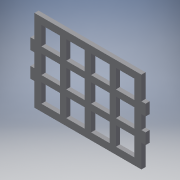
# Autodesk Inventor part: Top
Saved by Autodesk Inventor 2018 (Build 220112000, 112)
## iProperties
Created: 2017-10-30
Part Number: Top
Material: Polycarbonate, Clear
Document SubType Name: Modeling
Designer: xl0
Density: 1.2 g/cm^3
Appearance: Polycarbonate - Clear
Author: xl0
Autodesk Inventor part; units mm, degrees
ref_plane "YZ Plane" through (0, 0, 0) normal (1, 0, 0) x (0, 1, 0)
ref_plane "XZ Plane" through (0, 0, 0) normal (0, 1, 0) x (-1, 0, 0)
ref_plane "XY Plane" through (0, 0, 0) normal (0, 0, 1) x (1, 0, 0)
sketch "Sketch1" plane through (0, 0, 0) normal (0, 0, 1) x (1, 0, 0)
  line L0 (-38.75, 29.75) -> (38.75, 29.75)
  line L1 (38.75, 29.75) -> (38.75, -29.75)
  line L2 (38.75, -29.75) -> (-38.75, -29.75)
  line L3 (-38.75, -29.75) -> (-38.75, 29.75)
  line L4 (-33.75, 24.75) -> (-20.25, 24.75)
  line L5 (-20.25, 24.75) -> (-20.25, 11.25)
  line L6 (-20.25, 11.25) -> (-33.75, 11.25)
  line L7 (-33.75, 11.25) -> (-33.75, 24.75)
  line L8 (-2.25, 24.75) -> (-2.25, 11.25)
  line L9 (-15.75, 24.75) -> (-2.25, 24.75)
  line L10 (-15.75, 11.25) -> (-15.75, 24.75)
  line L11 (-2.25, 11.25) -> (-15.75, 11.25)
  line L12 (15.75, 24.75) -> (15.75, 11.25)
  line L13 (2.25, 24.75) -> (15.75, 24.75)
  line L14 (2.25, 11.25) -> (2.25, 24.75)
  line L15 (15.75, 11.25) -> (2.25, 11.25)
  line L16 (33.75, 24.75) -> (33.75, 11.25)
  line L17 (20.25, 24.75) -> (33.75, 24.75)
  line L18 (20.25, 11.25) -> (20.25, 24.75)
  line L19 (33.75, 11.25) -> (20.25, 11.25)
  line L20 (-20.25, 6.75) -> (-20.25, -6.75)
  line L21 (-33.75, 6.75) -> (-20.25, 6.75)
  line L22 (-33.75, -6.75) -> (-33.75, 6.75)
  line L23 (-20.25, -6.75) -> (-33.75, -6.75)
  line L24 (-2.25, 6.75) -> (-2.25, -6.75)
  line L25 (-15.75, 6.75) -> (-2.25, 6.75)
  line L26 (-15.75, -6.75) -> (-15.75, 6.75)
  line L27 (-2.25, -6.75) -> (-15.75, -6.75)
  line L28 (15.75, 6.75) -> (15.75, -6.75)
  line L29 (2.25, 6.75) -> (15.75, 6.75)
  line L30 (2.25, -6.75) -> (2.25, 6.75)
  line L31 (15.75, -6.75) -> (2.25, -6.75)
  line L32 (33.75, 6.75) -> (33.75, -6.75)
  line L33 (20.25, 6.75) -> (33.75, 6.75)
  line L34 (20.25, -6.75) -> (20.25, 6.75)
  line L35 (33.75, -6.75) -> (20.25, -6.75)
  line L36 (-20.25, -11.25) -> (-20.25, -24.75)
  line L37 (-33.75, -11.25) -> (-20.25, -11.25)
  line L38 (-33.75, -24.75) -> (-33.75, -11.25)
  line L39 (-20.25, -24.75) -> (-33.75, -24.75)
  line L40 (-2.25, -11.25) -> (-2.25, -24.75)
  line L41 (-15.75, -11.25) -> (-2.25, -11.25)
  line L42 (-15.75, -24.75) -> (-15.75, -11.25)
  line L43 (-2.25, -24.75) -> (-15.75, -24.75)
  line L44 (15.75, -11.25) -> (15.75, -24.75)
  line L45 (2.25, -11.25) -> (15.75, -11.25)
  line L46 (2.25, -24.75) -> (2.25, -11.25)
  line L47 (15.75, -24.75) -> (2.25, -24.75)
  line L48 (33.75, -11.25) -> (33.75, -24.75)
  line L49 (20.25, -11.25) -> (33.75, -11.25)
  line L50 (20.25, -24.75) -> (20.25, -11.25)
  line L51 (33.75, -24.75) -> (20.25, -24.75)
  line L52 (-38.75, 13) -> (-41.75, 13)
  line L53 (-41.75, 13) -> (-41.75, 5)
  line L54 (-41.75, 5) -> (-38.75, 5)
  line L55 (-38.75, -5) -> (-41.75, -5)
  line L56 (-41.75, -5) -> (-41.75, -13)
  line L57 (-41.75, -13) -> (-38.75, -13)
  line L58 (-22.2351, 9) -> (-45.0452, 9) construction
  line L59 (-22.7359, -9) -> (-44.2257, -9) construction
  line L60 (38.75, 13) -> (41.75, 13)
  line L61 (41.75, 13) -> (41.75, 5)
  line L62 (41.75, 5) -> (38.75, 5)
  line L63 (38.75, -5) -> (41.75, -5)
  line L64 (41.75, -5) -> (41.75, -13)
  line L65 (41.75, -13) -> (38.75, -13)
  point P0 (0, 0)
  point P1 (0, 29.75)
  point P2 (-38.75, 0)
  dimension "d0" = 13.5
  dimension "d1" = 5
  dimension "d2" = 5
  dimension "d5" = 18
  dimension "d8" = 18
  dimension "d11" = 5
  dimension "d12" = 5
  dimension "d13" = 8
  dimension "d14" = 3
  constraints: 132 end point, 9 horizontal, 9 perpendicular, 9 point on line, 5 collinear, 4 parallel, 3 equal length, 2 midpoint, 2 vertical, 1 horizontal alignment, 1 vertical alignment, 92 other
  measures "d0" distance of L5.end L6.end
  measures "d1" distance between parallel lines of L0 L4
  measures "d2" distance between parallel lines of L3 L7
  measures "d5" distance of L4.end L8.start
  measures "d8" distance of L4.end L20.start
  measures "d11" distance between parallel lines of L16 L1
  measures "d12" distance between parallel lines of L2 L51
  measures "d13" distance of L52.end L53.end
  measures "d14" distance between parallel lines of L3 L53
extrude "Extrusion1" add sketch "Sketch1" along normal blind 3
equation "\"d2\" = d1"
equation "\"d11\" = d1"
equation "\"d12\" = d1"
body "Solid1"
